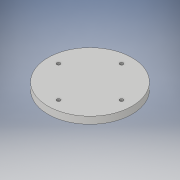
# Autodesk Inventor part: CrankAttachment_SBail
Saved by Autodesk Inventor 2019 (Build 230136000, 136)
## iProperties
Created: 2019-05-29
Part Number: CrankAttachment_SBail
Material: Generic
Document SubType Name: Modeling
Designer: samson.bailor
Density: 1 g/cm^3
Appearance: Default
Author: samson.bailor
Autodesk Inventor part; units mm, degrees
ref_plane "YZ Plane" through (0, 0, 0) normal (1, 0, 0) x (0, 1, 0)
ref_plane "XZ Plane" through (0, 0, 0) normal (0, 1, 0) x (-1, 0, 0)
ref_plane "XY Plane" through (0, 0, 0) normal (0, 0, 1) x (1, 0, 0)
sketch "Sketch1" plane through (0, 0, 0) normal (0, 1, 0) x (-1, 0, 0)
  circle A0 centre (0, 0) radius 12.7
  circle A1 centre (0, 0) radius 9.652
  circle A2 centre (0, 0) radius 38.1
  dimension "d0" = 25.4
  dimension "d1" = 19.304
  dimension "d2" = 76.2
  constraints: 3 centre point, 3 coincident
  measures "d0" diameter of A0
  measures "d1" diameter of A1
  measures "d2" diameter of A2
extrude "Extrusion1" add sketch "Sketch1" along normal blind 6.35
sketch "Sketch2" plane through (0, 6.35, 0) normal (0, 1, 0) x (1, 0, 0)
  circle A0 centre (0, 0) radius 38.1
  constraints: 1 centre point, 1 coincident
extrude "Extrusion2" add sketch "Sketch2" along normal blind 2.54
sketch "Sketch3" plane through (0, 0, 0) normal (0, -1, 0) x (1, 0, 0)
  circle A0 centre (0, 0) radius 38.1
  constraints: 1 centre point, 1 coincident
extrude "Extrusion3" cut sketch "Sketch3" against normal blind 2.54
sketch "Sketch4" plane through (0, 2.54, 0) normal (0, -1, 0) x (1, 0, 0)
  circle A0 centre (0, 0) radius 19.05
  circle A1 centre (0, 0) radius 12.7
  circle A2 centre (0, 0) radius 9.652
  dimension "d9" = 38.1
  constraints: 3 centre point, 3 coincident
  measures "d9" diameter of A0
extrude "Extrusion4" add sketch "Sketch4" along normal blind 6.35
sketch "Sketch5" plane through (0, 2.54, 0) normal (0, -1, 0) x (1, 0, 0)
  circle A0 centre (0, 0) radius 38.1 projected
  line L0 (38.1, 0) -> (19.05, 0)
  circle A1 centre (0, 0) radius 19.05 projected
  line L1 (0, 18.9941) -> (0, 38.0123)
  line L2 (-19.05, 0) -> (-38.1, 0)
  line L3 (0, -19.05) -> (0, -38.1)
  circle A2 centre (0, 28.5032) radius 1.5875
  circle A3 centre (28.575, 0) radius 1.5875
  circle A4 centre (0, -28.575) radius 1.5875
  circle A5 centre (-28.575, 0) radius 1.5875
  dimension "d12" = 3.175
  dimension "d13" = 3.175
  dimension "d14" = 3.175
  dimension "d15" = 3.175
  constraints: 8 end point, 6 point on circle, 4 centre point, 4 midpoint, 2 horizontal, 1 perpendicular, 1 vertical
  measures "d12" diameter of A2
  measures "d13" diameter of A3
  measures "d14" diameter of A4
  measures "d15" diameter of A5
extrude "Extrusion5" cut sketch "Sketch5" against normal blind 6.35 contours A2 L1 | L1 A2 | A3 L0 | L0 A3 | A5 L2 | L2 A5 | A4 L3 | L3 A4
body "Solid1"
